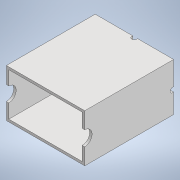
# Autodesk Inventor part: Lower Support
Saved by Autodesk Inventor 2022 (Build 260153000, 153)
## iProperties
Created: 2021-11-30
Part Number: Lower Support
Material: Generic
Document SubType Name: Modeling
Designer: efred
Density: 1 g/cm^3
Appearance: Default
Author: efred
Autodesk Inventor part; units mm, degrees
ref_plane "YZ Plane" through (0, 0, 0) normal (1, 0, 0) x (0, 1, 0)
ref_plane "XZ Plane" through (0, 0, 0) normal (0, 1, 0) x (-1, 0, 0)
sketch "Sketch1" plane through (0, 0, 0) normal (0, 0, 1) x (1, 0, 0)
  line L0 (320.4, 0) -> (420.4, 0) construction
  line L1 (420.4, 0) -> (420.4, -10) construction
  line L2 (320.4, -10) -> (420.4, -10) construction
  line L3 (320.4, 0) -> (320.4, -10) construction
  line L4 (409.3, 0.1) -> (409.3, 50.1) construction
  line L5 (420.4, 0.1) -> (409.3, 0.1) construction
  line L6 (420.4, 50.1) -> (420.4, 0.1) construction
  line L7 (409.3, 50.1) -> (420.4, 50.1) construction
  line L8 (420.5, 50.2) -> (409.2, 50.2)
  line L9 (409.2, 50.2) -> (409.2, 35.3)
  line L10 (409.2, 35.3) -> (404.07, 35.3)
  line L11 (404.07, 35.3) -> (404.07, 7.3)
  line L12 (402.07, 5.3) -> (389.1, 5.3)
  line L13 (389.1, 5.3) -> (389.1, 0.1)
  line L14 (389.1, 0.1) -> (320.3, 0.1)
  line L15 (320.3, 0.1) -> (320.3, -10.1)
  line L16 (320.3, -10.1) -> (420.5, -10.1)
  line L17 (420.5, -10.1) -> (420.5, 50.2)
  arc A0 (402.07, 5.3) -> (404.07, 7.3) centre (402.07, 7.3) ccw
  line L18 (315.3, 5.1) -> (384.1, 5.1)
  line L19 (384.1, 5.1) -> (384.1, 10.3)
  line L20 (384.1, 10.3) -> (399.07, 10.3)
  line L21 (399.07, 10.3) -> (399.07, 40.3)
  line L22 (399.07, 40.3) -> (404.2, 40.3)
  line L23 (404.2, 40.3) -> (404.2, 55.2)
  line L24 (404.2, 55.2) -> (425.5, 55.2)
  line L25 (425.5, 55.2) -> (425.5, -15.1)
  line L26 (425.5, -15.1) -> (315.3, -15.1)
  line L27 (315.3, -15.1) -> (315.3, 5.1)
  line L28 (404.2, 7.2) -> (404.2, 35.2) projected
  arc A1 (402.2, 5.2) -> (404.2, 7.2) centre (402.2, 7.2) ccw projected
  line L29 (389.2, 5.2) -> (402.2, 5.2) projected
  line L30 (389.2, 0.2) -> (389.2, 5.2) projected
  line L31 (409.2, 0.2) -> (389.2, 0.2) projected
  line L32 (409.2, 35.2) -> (409.2, 0.2) projected
  line L33 (404.2, 35.2) -> (409.2, 35.2) projected
  point P0 (0, 0)
  dimension "d0" = 0.1
  dimension "d1" = 0.1
  dimension "d2" = 0.1
  dimension "d6" = 2
  dimension "d8" = 0.1
  dimension "d9" = 0.1
  dimension "d10" = 0.1
  dimension "d11" = 5
  dimension "d72" = 0.1
  dimension "d73" = 0.1
  dimension "d74" = 0.13
  dimension "d75" = 0.1
  constraints: 40 end point, 14 perpendicular, 2 point on circle, 2 tangent, 1 centre point, 1 horizontal, 1 parallel, 1 vertical, 9 other
  measures "d0" distance between parallel lines of L7 L8
  measures "d1" distance between parallel lines of L6 L17
  measures "d2" distance between parallel lines of L4 L9
  measures "d6" radius of A0
  measures "d8" distance between parallel lines of L0 L14
  measures "d9" distance between parallel lines of L3 L15
  measures "d10" distance between parallel lines of L2 L16
  measures "d11" distance between parallel lines of L14 L18
  measures "d72" distance between parallel lines of L30 L13
  measures "d73" distance between parallel lines of L29 L12
  measures "d74" distance between parallel lines of L28 L11
  measures "d75" distance between parallel lines of L33 L10
extrude "Extrusion1" add sketch "Sketch1" against normal blind 12 contours L18 L19 L20 L21 L22 L23 L24 L25 L26 L27
sketch "Sketch4" plane through (0, 0, 0) normal (0, 0, 1) x (1, 0, 0)
  line L0 (194.6531, 87.1) -> (247.6531, 87.1) projected
  line L1 (315.3, 82.1) -> (475, 82.1)
  line L2 (475, -15.1) -> (315.3, -15.1)
  line L3 (315.3, -15.1) -> (315.3, 82.1)
  line L4 (315.3, -15.1) -> (425.5, -15.1) projected
  line L5 (315.3, 5.1) -> (315.3, -15.1) projected
  line L6 (475, 9.2) -> (475, 65.2) projected
  line L7 (475, -15.1) -> (475, 82.1)
  point P0 (0, 0)
  dimension "d66" = 5
  constraints: 8 end point, 3 collinear, 1 horizontal, 1 parallel, 1 vertical
  measures "d66" distance between parallel lines of L0 L1
extrude "Extrusion4" add sketch "Sketch4" along normal blind 169
sketch "Sketch5" plane through (0, 0, 169) normal (0, 0, 1) x (1, 0, 0)
  line L0 (315.3, 82.1) -> (315.3, -15.1) projected
  line L1 (315.3, -15.1) -> (475, -15.1) projected
  line L2 (475, -15.1) -> (475, 82.1) projected
  line L3 (475, 82.1) -> (315.3, 82.1) projected
  line L4 (320.3, 77.1) -> (320.3, -10.1)
  line L5 (320.3, -10.1) -> (470, -10.1)
  line L6 (470, -10.1) -> (470, 77.1)
  line L7 (470, 77.1) -> (320.3, 77.1)
  point P0 (0, 0)
  dimension "d26" = 5
  constraints: 8 end point, 3 other
  measures "d26" distance between parallel lines of L3 L7
extrude "Extrusion5" cut sketch "Sketch5" against normal blind 160 contours L7 L6 L5 L4
sketch "Sketch6" plane through (0, 0, 0) normal (0, 0, -1) x (-1, 0, 0)
  line L0 (-384.1, 5.1) -> (-315.3, 5.1) projected
  line L1 (-315.3, 82.1) -> (-315.3, 5.1) projected
  line L2 (-475, 82.1) -> (-315.3, 82.1) projected
  line L3 (-475, -15.1) -> (-475, 82.1) projected
  line L4 (-425.5, -15.1) -> (-475, -15.1) projected
  line L5 (-425.5, -15.1) -> (-425.5, 55.2) projected
  line L6 (-425.5, 55.2) -> (-404.2, 55.2) projected
  line L7 (-404.2, 55.2) -> (-404.2, 40.3) projected
  line L8 (-404.2, 40.3) -> (-399.07, 40.3) projected
  line L9 (-399.07, 40.3) -> (-399.07, 10.3) projected
  line L10 (-399.07, 10.3) -> (-384.1, 10.3) projected
  line L11 (-384.1, 10.3) -> (-384.1, 5.1) projected
  point P0 (0, 0)
extrude "Extrusion6" add sketch "Sketch6" along normal up to surface (12 mm away)
sketch "Sketch7" plane through (315.3, 82.1, 169) normal (0, 1, 0) x (1, 0, 0)
  circle A0 centre (81.4, 179.1) radius 5
  circle A1 centre (36.4, 176.6) radius 2.5 construction
  circle A2 centre (51.4, 176.6) radius 2.5 construction
  circle A3 centre (21.4, 176.6) radius 2.5 construction
  circle A4 centre (66.4, 176.6) radius 2.5 construction
  circle A5 centre (81.4, 179.1) radius 2.5 construction
  circle A6 centre (81.4, 194.1) radius 2.5 construction
  circle A7 centre (81.4, 209.1) radius 2.5 construction
  line L0 (5.1, 169.1) -> (5.1, 312.15) construction
  line L1 (5.1, 312.15) -> (105.1, 312.15) construction
  line L2 (105.1, 312.15) -> (105.1, 169.1) construction
  line L3 (105.1, 169.1) -> (5.1, 169.1) construction
  circle A8 centre (10.1, 282.25) radius 2.15 construction
  circle A9 centre (10.1, 302.15) radius 2.15 construction
  circle A10 centre (88.9, 302.15) radius 2.15 construction
  circle A11 centre (88.9, 282.25) radius 2.15 construction
  circle A12 centre (99.55, 189.1) radius 2.65 construction
  circle A13 centre (99.55, 209.1) radius 2.65 construction
  circle A14 centre (99.55, 229.1) radius 2.65 construction
  circle A15 centre (99.55, 249.1) radius 2.65 construction
  point P0 (-315.3, 169)
  dimension "d71" = 10
  constraints: 2 coincident, 1 centre point
  measures "d71" diameter of A0
ref_plane "Work Plane2" through (389.2, 5.1, -50.1) normal (0, 1, 0) x (0, 0, 1)
extrude "Extrusion7" cut sketch "Sketch7" against normal through all
sketch "Sketch8" plane through (404.07, 7.3, -12) normal (1, 0, 0) x (0, 0, -1)
  circle A0 centre (-1.9, 21.9) radius 2.5 construction
  circle A1 centre (-1.9, 21.9) radius 2.5 construction
  circle A2 centre (-1.9, 21.9) radius 5
  point P0 (-12, -7.3)
  dimension "d34" = 10
  constraints: 1 centre point, 1 coincident
  measures "d34" diameter of A2
extrude "Extrusion8" cut sketch "Sketch8" along normal through all both and the other way through all
sketch "Sketch9" plane through (315.3, -15.1, 169) normal (0, -1, 0) x (1, 0, 0)
  circle A0 centre (81.4, -179.1) radius 3.0567 construction
  line L0 (107.734, -169) -> (7.734, -169) construction
  circle A1 centre (66.4, -176.5) radius 2.65
  circle A2 centre (51.4, -176.5) radius 2.65
  circle A3 centre (36.4, -176.5) radius 2.65
  circle A4 centre (21.4, -176.5) radius 2.65
  line L1 (105.2, -169) -> (5, -169) construction
  circle A5 centre (81.4, -179.1) radius 2.5 construction
  point P0 (-315.3, -169)
  dimension "d37" = 5.3
  dimension "d38" = 7.5
  dimension "d39" = 15
  dimension "d42" = 15
  constraints: 5 centre point, 2 end point, 1 coincident, 1 collinear, 1 horizontal, 6 other
  measures "d37" diameter of A1
  measures "d38" distance from line of L0 A1.centre
  measures "d39" horizontal distance of A0.centre A1.centre
  measures "d42" distance of A1.centre A2.centre
extrude "Extrusion9" cut sketch "Sketch9" against normal blind 45
sketch "Sketch10" plane through (475, -15.1, 169) normal (1, 0, 0) x (0, 0, -1)
  circle A0 centre (0, 48.6) radius 20
  line L0 (0, 48.6) -> (279.056, 48.6) construction
  line L1 (0, 0) -> (0, 97.2) projected
  point P0 (169, 15.1)
  dimension "d49" = 40
  constraints: 2 end point, 2 midpoint, 1 centre point, 1 horizontal, 1 point on line
  measures "d49" diameter of A0
extrude "Extrusion10" cut sketch "Sketch10" against normal through all
fillet "Fillet2" radius 10 4 edges at (395.15, -10.1, 9) (470, 33.5, 9) (395.15, 77.1, 9) (320.3, 33.5, 9)
sketch "Sketch13" plane through (315.3, -15.1, 169) normal (0, -1, 0) x (1, 0, 0)
  line L0 (0, 0) -> (159.7, 0) projected
  circle A0 centre (79.7, 0) radius 20
  point P0 (-315.3, -169)
  point P1 (99.7, 0)
  point P2 (59.7, 0)
  dimension "d77" = 40
  dimension "d78" = 80
  constraints: 1 centre point, 1 point on line
  measures "d77" diameter of A0
  measures "d78" distance of L0.end A0.centre
extrude "Extrusion13" cut sketch "Sketch13" against normal up to next contours L0 A0 picked at (83.4871, -5.4866)
body "Solid1"
